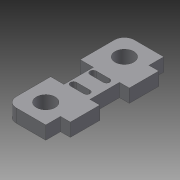
# Autodesk Inventor part: Carriage_Joint_Frame
Saved by Autodesk Inventor 2014 (Build 180170000, 170)
## iProperties
Created: 2014-08-27
Part Number: Carriage_Joint_Frame
Material: Generic
Document SubType Name: Modeling
Designer: ThatOtherGuy
Density: 1 g/cm^3
Appearance: Default
Author: ThatOtherGuy
Autodesk Inventor part; units mm, degrees
ref_plane "YZ Plane" through (0, 0, 0) normal (1, 0, 0) x (0, 1, 0)
ref_plane "XZ Plane" through (0, 0, 0) normal (0, 1, 0) x (-1, 0, 0)
ref_plane "XY Plane" through (0, 0, 0) normal (0, 0, 1) x (1, 0, 0)
sketch "Sketch1" plane through (0, 0, 0) normal (0, 0, 1) x (1, 0, 0)
  line L0 (0, 0) -> (0, 60)
  line L1 (0, 60) -> (20, 60)
  line L2 (20, 60) -> (20, 52.5)
  line L3 (20, 52.5) -> (25, 52.5)
  line L4 (25, 52.5) -> (25, 37.5)
  line L5 (25, 37.5) -> (20, 37.5)
  line L6 (20, 37.5) -> (20, 22.5)
  line L7 (20, 22.5) -> (25, 22.5)
  line L8 (25, 22.5) -> (25, 7.5)
  line L9 (25, 7.5) -> (20, 7.5)
  line L10 (20, 7.5) -> (20, 0)
  line L11 (20, 0) -> (0, 0)
  circle A0 centre (10, 10) radius 4.75
  circle A1 centre (10, 50) radius 4.75
  circle A2 centre (5, 41.25) radius 1.59
  circle A3 centre (12.5, 30) radius 1.59
  line L12 (7.5, 36.5875) -> (17.5, 36.5875)
  line L13 (17.5, 36.5875) -> (17.5, 33.4125)
  line L14 (17.5, 33.4125) -> (7.5, 33.4125)
  line L15 (7.5, 33.4125) -> (7.5, 36.5875)
  line L16 (7.5, 26.5875) -> (17.5, 26.5875)
  line L17 (17.5, 26.5875) -> (17.5, 23.4125)
  line L18 (17.5, 23.4125) -> (7.5, 23.4125)
  line L19 (7.5, 23.4125) -> (7.5, 26.5875)
  line L20 (9.0875, 35) -> (15.9125, 35) construction
  line L21 (9.0875, 33.4125) -> (15.9125, 33.4125)
  line L22 (15.9125, 36.5875) -> (9.0875, 36.5875)
  arc A4 (9.0875, 36.5875) -> (9.0875, 33.4125) centre (9.0875, 35) ccw
  arc A5 (15.9125, 33.4125) -> (15.9125, 36.5875) centre (15.9125, 35) ccw
  line L23 (9.0875, 25) -> (15.9125, 25) construction
  line L24 (9.0875, 23.4125) -> (15.9125, 23.4125)
  line L25 (15.9125, 26.5875) -> (9.0875, 26.5875)
  arc A6 (9.0875, 26.5875) -> (9.0875, 23.4125) centre (9.0875, 25) ccw
  arc A7 (15.9125, 23.4125) -> (15.9125, 26.5875) centre (15.9125, 25) ccw
  point P0 (12.5, 35)
  point P1 (12.5, 25)
  point P2 (20, 30)
  dimension "d0" = 15
  dimension "d1" = 60
  dimension "d2" = 20
  dimension "d3" = 5
  dimension "d6" = 9.5
  dimension "d7" = 40
  dimension "d8" = 10
  dimension "d9" = 10
  dimension "d11" = 10
  dimension "d12" = 10
  dimension "d25" = 3.18
  dimension "d26" = 15
  dimension "d29" = 2.5
  dimension "d30" = 3.175
  dimension "d33" = 10
  dimension "d34" = 10
  dimension "d35" = 5
  dimension "d36" = 7.5
  dimension "d37" = 11.25
  constraints: 60 end point, 18 parallel, 16 tangent, 8 centre point, 8 equal length, 8 point on circle, 3 midpoint, 3 perpendicular, 2 equal radius, 2 horizontal, 1 collinear, 1 horizontal alignment, 1 vertical, 1 vertical alignment
  measures "d0" distance of L5.end L6.end
  measures "d1" distance of L0.start L0.end
  measures "d2" distance of L10.end L0.start
  measures "d3" distance of L4.end L5.end
  measures "d6" diameter of A1
  measures "d7" distance of A0.centre A1.centre
  measures "d8" distance from line of A1.centre L1
  measures "d9" distance from line of L11 A0.centre
  measures "d11" distance from line of L2 A1.centre
  measures "d12" distance from line of A1.centre L0
  measures "d25" diameter of A3
  measures "d26" distance from line of L6 A2.centre
  measures "d29" distance between parallel lines of L6 L17
  measures "d30" distance of L16.end L17.end
  measures "d33" distance of L12.start L12.end
  measures "d34" distance between parallel lines of L23 L20
  measures "d35" distance from line of L20 point (20, 30)
  measures "d36" distance from line of L6 A3.centre
  measures "d37" vertical distance of A2.centre A3.centre
extrude "Extrusion1" add sketch "Sketch1" along normal blind 6.731 contours L0 L1 L2 L3 L4 L5 L6 L7 L8 L9 L10 L11 | A2 | A3 | L12 A4 L15 | L12 A5 L14 A4 | A4 L14 L15 | L12 L13 A5 | L13 L14 A5 | L16 A6 L19 | L16 A7 L18 A6 | A6 L18 L19 | L16 L17 A7 | L17 L18 A7
sketch "Sketch2" plane through (0, 0, 0) normal (0, 0, -1) x (-1, 0, 0)
  line L0 (0, 0) -> (-20, 0) projected
  line L1 (0, 60) -> (0, 0) projected
  line L2 (-20, 22.5) -> (-20, 37.5) projected
  line L3 (0, 22.5) -> (-6.731, 22.5)
  line L4 (-6.731, 22.5) -> (-6.731, 37.5)
  line L5 (-6.731, 37.5) -> (0, 37.5)
  line L6 (0, 37.5) -> (0, 22.5)
  line L7 (-9.0875, 25) -> (-15.9125, 25) construction
  line L8 (-9.0875, 26.5875) -> (-15.9125, 26.5875)
  line L9 (-15.9125, 23.4125) -> (-9.0875, 23.4125)
  arc A0 (-9.0875, 23.4125) -> (-9.0875, 26.5875) centre (-9.0875, 25) ccw
  arc A1 (-15.9125, 26.5875) -> (-15.9125, 23.4125) centre (-15.9125, 25) ccw
  line L10 (-9.0875, 35) -> (-15.9125, 35) construction
  line L11 (-9.0875, 36.5875) -> (-15.9125, 36.5875)
  line L12 (-15.9125, 33.4125) -> (-9.0875, 33.4125)
  arc A2 (-9.0875, 33.4125) -> (-9.0875, 36.5875) centre (-9.0875, 35) ccw
  arc A3 (-15.9125, 36.5875) -> (-15.9125, 33.4125) centre (-15.9125, 35) ccw
  point P0 (0, 30)
  point P1 (0, 30)
  point P2 (-12.5, 25)
  point P3 (-12.5, 35)
  dimension "d38" = 6.731
  dimension "d39" = 15
  dimension "d40" = 10
  dimension "d41" = 3.175
  dimension "d42" = 6.825
  dimension "d43" = 2.5
  dimension "d44" = 5
  constraints: 24 end point, 8 point on circle, 8 tangent, 7 parallel, 4 centre point, 4 midpoint, 1 coincident, 1 equal radius, 1 horizontal, 1 perpendicular, 1 point on line, 1 vertical alignment
  measures "d38" distance of L4.end L5.end
  measures "d39" distance of L3.end L4.end
  measures "d40" distance between parallel lines of L10 L7
  measures "d41" distance between parallel lines of L8 L9
  measures "d42" distance of L7.start L7.end
  measures "d43" distance edge to line of A1 L2
  measures "d44" distance from line of point (0, 30) L10
extrude "Extrusion2" cut sketch "Sketch2" against normal up to next
fillet "Fillet1" radius 5 2 edges at (0, 60, 3.3655) (0, 0, 3.3655)
equation "\"d6\" = MAGDIA"
equation "\"d8\" = d9"
equation "\"d11\" = d12"
equation "\"d35\" = 0.5 * d34"
equation "\"d4\" = THICKB"
equation "\"d38\" = THICKB"
equation "\"d44\" = 0.5 * d40"
equation "\"THICKA\" = 3.175"
equation "\"THICKB\" = 6.731"
equation "\"THICKC\" = 12.7"
equation "\"MAGDIA\" = 9.5"
equation "\"BALLDIA\" = 12"
equation "\"THICKPLY\" = 5"
body "Solid1"
